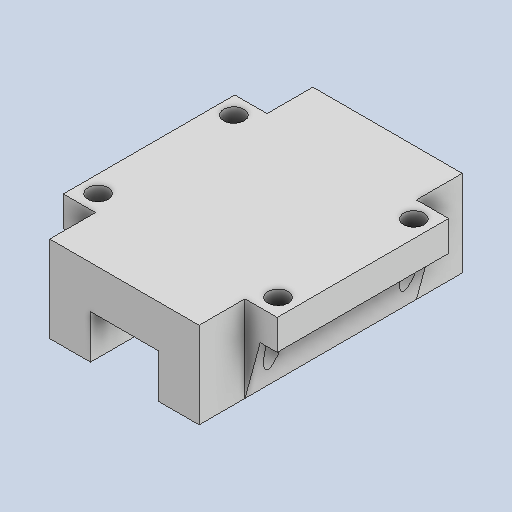
# Autodesk Inventor part: HGW20CC_Slider
Saved by Autodesk Inventor 2023 (Build 270158000, 158)
## iProperties
Created: 2022-05-01
Part Number: HGW20CC_Slider
Material: Generic
Document SubType Name: Modeling
Designer: plebbb
Density: 1 g/cm^3
Appearance: Default
Mass: 77.6376 g
Surface Area: 170.382 cm^2
Volume: 77.6376 cm^3
Author: plebbb
Autodesk Inventor part; units mm, degrees
ref_plane "YZ Plane" through (0, 0, 0) normal (1, 0, 0) x (0, 1, 0)
ref_plane "XZ Plane" through (0, 0, 0) normal (0, 1, 0) x (-1, 0, 0)
ref_plane "XY Plane" through (0, 0, 0) normal (0, 0, 1) x (1, 0, 0)
sketch "Sketch1" plane through (0, 0, 0) normal (0, 0, 1) x (1, 0, 0)
  line L0 (0, 0) -> (63, 0)
  line L1 (53.5, -25.4) -> (41.5, -25.4)
  line L2 (41.5, -25.4) -> (41.5, -12.5)
  line L3 (41.5, -12.5) -> (21.5, -12.5)
  line L4 (21.5, -12.5) -> (21.5, -25.4)
  line L5 (0, 0) -> (0, -8.9)
  line L6 (0, -8.9) -> (5, -8.9)
  line L7 (5, -8.9) -> (9.5, -25.4)
  line L8 (9.5, -25.4) -> (21.5, -25.4)
  line L9 (53.5, -25.4) -> (58, -8.9)
  line L10 (58, -8.9) -> (63, -8.9)
  line L11 (63, -8.9) -> (63, 0)
  point P0 (31.5, -12.5)
  point P1 (31.5, 0)
  dimension "d0" = 63
  dimension "d1" = 25.4
  dimension "d4" = 21.5
  dimension "d5" = 8.9
  dimension "d6" = 12.9
  dimension "d7" = 12
  dimension "d8" = 5
  constraints: 24 end point, 7 perpendicular, 3 equal length, 2 horizontal, 2 midpoint, 1 coincident, 1 point on line, 1 vertical, 1 vertical alignment
  measures "d0" distance of L0.start L0.end
  measures "d1" distance from line of point (0, 0) L8
  measures "d4" distance between parallel lines of L5 L4
  measures "d5" distance of L0.start L5.end
  measures "d6" distance between parallel lines of L8 L3
  measures "d7" distance of L7.end L4.end
  measures "d8" distance of L5.end L6.end
extrude "Extrusion1" add sketch "Sketch1" along normal blind 50.5
sketch "Sketch2" plane through (0, 0, 50.5) normal (0, 0, 1) x (1, 0, 0)
  line L0 (21.5, -25.4) -> (21.5, -12.5) projected
  line L1 (41.5, -12.5) -> (41.5, -25.4) projected
  line L2 (9.5, -25.4) -> (21.5, -25.4) projected
  line L3 (41.5, -25.4) -> (53.5, -25.4) projected
  line L4 (9.5, -25.4) -> (9.5, 0)
  line L5 (9.5, 0) -> (53.5, 0)
  line L6 (53.5, 0) -> (53.5, -25.4)
  line L7 (21.5, -12.5) -> (41.5, -12.5) projected
  point P0 (0, 0)
  point P1 (31.5, 0)
  constraints: 6 end point, 3 perpendicular, 1 horizontal alignment, 1 midpoint
extrude "Extrusion2" add sketch "Sketch2" along normal blind 13.5 and the other way blind 64
sketch "Sketch3" plane through (63, 0, 50.5) normal (0, 1, 0) x (1, 0, 0)
  circle A0 centre (-58, 5.25) radius 3
  circle A1 centre (-58, 45.25) radius 3
  circle A2 centre (-5, 5.25) radius 3
  circle A3 centre (-5, 45.25) radius 3
  line L0 (-58, 5.25) -> (-5, 5.25) construction
  line L1 (-5, 5.25) -> (-5, 45.25) construction
  line L2 (-5, 45.25) -> (-58, 45.25) construction
  line L3 (-58, 45.25) -> (-58, 5.25) construction
  line L4 (-53.5, 64) -> (-9.5, 64) projected
  line L5 (-63, 50.5) -> (-63, 0) projected
  point P0 (-31.5, 64)
  point P1 (-31.5, 45.25)
  point P2 (-58, 25.25)
  point P3 (-63, 25.25)
  dimension "d15" = 6
  dimension "d16" = 40
  dimension "d17" = 53
  constraints: 8 end point, 4 centre point, 4 midpoint, 3 coincident, 3 equal radius, 2 parallel, 1 horizontal, 1 horizontal alignment, 1 perpendicular, 1 vertical alignment
  measures "d15" diameter of A0
  measures "d16" distance of L2.end L0.start
  measures "d17" distance of L1.end L2.end
extrude "Extrusion3" cut sketch "Sketch3" against normal blind 34.5
body "Solid1"
